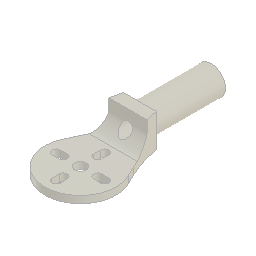
Motor-Arm Adaptor (Autodesk Fusion 360 design; units mm, degrees)
Autodesk Fusion 360 part; units mm, degrees
note: some values were not read from the file. Chosen so that the rebuilt part matches the saved one: which pieces of a blend or face edit are solid.
sketch "Sketch1" plane through (0, 0, 0) normal (0, 1, 0) x (1, 0, 0)
  line L0 (0, 0) -> (14, 0)
  line L1 (14, 0) -> (14, -14)
  line L2 (14, -14) -> (0, -14)
  line L3 (0, -14) -> (0, 0)
  dimension "d1" = 14
  dimension "d2" = 14
  constraint horizontal L0
  constraint vertical L1
  constraint horizontal L2
  constraint vertical L3
  constraint coincident L0.start L3.end
  measures "d1" distance of L0.start L0.end
  measures "d2" distance of L0.start L2.end
extrude "Extrude1" add sketch "Sketch1" along normal blind 5
sketch "Sketch2" plane through (0, 5, 0) normal (0, 1, 0) x (-1, 0, 0)
  line L0 (0, 14) -> (-14, 14)
  line L1 (-14, 14) -> (-14, 0)
  line L2 (-14, 0) -> (0, 0)
  line L3 (0, 0) -> (0, 14)
  circle A0 centre (-7, 7) radius 6
  circle A1 centre (-7, 7) radius 2.5
  dimension "d5" = 12
  dimension "d6" = 5
  constraint concentric A0 A1
  measures "d5" diameter of A0
  measures "d6" diameter of A1
extrude "Extrude2" cut sketch "Sketch2" against normal blind 11 contours A1
extrude "Extrude3" add sketch "Sketch2" along normal blind 30 contours A0
sketch "Sketch3" plane through (0, 0, 0) normal (0, 0, 1) x (1, 0, 0)
  line L0 (7, 5) -> (7, -35) construction
  circle A0 centre (7, -20) radius 15
  line L1 (14, 0) -> (0, 0)
  line L2 (0, 0) -> (-6.5078, -13.4777)
  line L3 (14, 0) -> (20.5078, -13.4777)
  circle A1 centre (7, -20) radius 2.5
  line L4 (-8, -20) -> (22, -20) construction
  line L5 (-3.25, -18.25) -> (-0.25, -18.25)
  line L6 (-0.25, -18.25) -> (-0.25, -21.75) construction
  line L7 (-0.25, -21.75) -> (-3.25, -21.75)
  line L8 (-3.25, -21.75) -> (-3.25, -18.25) construction
  arc A2 (-3.25, -18.25) -> (-3.25, -21.75) centre (-3.25, -20) ccw
  arc A3 (-0.25, -21.75) -> (-0.25, -18.25) centre (-0.25, -20) ccw
  line L9 (5.25, -30.25) -> (5.25, -27.25)
  arc A4 (5.25, -30.25) -> (8.75, -30.25) centre (7, -30.25) ccw
  line L10 (8.75, -27.25) -> (8.75, -30.25)
  arc A5 (8.75, -27.25) -> (5.25, -27.25) centre (7, -27.25) ccw
  line L11 (17.25, -21.75) -> (14.25, -21.75)
  arc A6 (17.25, -21.75) -> (17.25, -18.25) centre (17.25, -20) ccw
  line L12 (14.25, -18.25) -> (17.25, -18.25)
  arc A7 (14.25, -18.25) -> (14.25, -21.75) centre (14.25, -20) ccw
  line L13 (8.75, -9.75) -> (8.75, -12.75)
  arc A8 (8.75, -9.75) -> (5.25, -9.75) centre (7, -9.75) ccw
  line L14 (5.25, -12.75) -> (5.25, -9.75)
  arc A9 (5.25, -12.75) -> (8.75, -12.75) centre (7, -12.75) ccw
  dimension "d11" = 30
  dimension "d12" = 20
  dimension "d13" = 5
  dimension "d14" = 3.5
  dimension "d16" = 1.75
  dimension "d18" = 3
  dimension "d20" = 4.75
  dimension "d23" = 360
  constraint vertical L0
  constraint coincident L0 A0.centre
  constraint coincident L1.end L2.start
  constraint coincident A0 L2.end
  constraint tangent A0 L2
  constraint coincident L1.start L3.start
  constraint coincident A0 L3.end
  constraint tangent A0 L3
  constraint concentric A0 A1
  constraint coincident L0.end A0
  constraint coincident A0 L4.start
  constraint coincident A0 L4.end
  constraint perpendicular L0 L4
  constraint horizontal L5
  constraint vertical L6
  constraint horizontal L7
  constraint vertical L8
  constraint midpoint L8 A2.centre
  constraint midpoint L6 A3.centre
  constraint coincident A0.centre L4
  measures "d11" diameter of A0
  measures "d12" distance of A0.centre L1
  measures "d13" diameter of A1
  measures "d14" distance of L5.start L7.end
  measures "d16" distance of L4 L7
  measures "d18" distance of L5.start L5.end
  measures "d20" distance of L4.start A2.centre
extrude "Extrude4" add sketch "Sketch3" along normal blind 3
fillet "Fillet1" radius 6.25 tangency weight 0.5 1 edges at (7, 0, 3)
fillet "Fillet2" radius 50 2 edges at (14, 0, 4.625) (0, 0, 4.625)
equation "d12 = d11 / 2 + 5 mm"
equation "d16 = 0.5 * d14"
equation "d20 = ( ( d11 - d13 ) / 2 - d18 ) / 2"
named bodies: "Motor Arm Adaptor"
